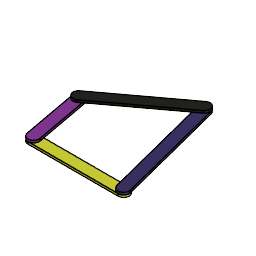
four_bar_linkage (Autodesk Fusion 360 design; units mm, degrees)
Autodesk Fusion 360 part; units mm, degrees
sketch "Sketch1" plane through (0, 0, 0) normal (0, 0, 1) x (1, 0, 0)
  line L0 (0, -5) -> (50, -5)
  arc A0 (50, -5) -> (50, 5) centre (50, 0) ccw
  line L1 (50, 5) -> (0, 5)
  arc A1 (0, 5) -> (0, -5) centre (0, 0) ccw
  line L2 (0, 0) -> (50, 0) construction
  line L3 (0, -25) -> (80, -25)
  arc A2 (80, -25) -> (80, -15) centre (80, -20) ccw
  line L4 (80, -15) -> (0, -15)
  arc A3 (0, -15) -> (0, -25) centre (0, -20) ccw
  line L5 (0, -20) -> (80, -20) construction
  line L6 (0, -45) -> (80, -45)
  arc A4 (80, -45) -> (80, -35) centre (80, -40) ccw
  line L7 (80, -35) -> (0, -35)
  arc A5 (0, -35) -> (0, -45) centre (0, -40) ccw
  line L8 (0, -40) -> (80, -40) construction
  line L9 (0, -65) -> (100, -65)
  arc A6 (100, -65) -> (100, -55) centre (100, -60) ccw
  line L10 (100, -55) -> (0, -55)
  arc A7 (0, -55) -> (0, -65) centre (0, -60) ccw
  line L11 (0, -60) -> (100, -60) construction
  dimension "d1" = 10
  dimension "d2" = 10
  dimension "d3" = 10
  dimension "d4" = 10
  constraint tangent L0 A0
  constraint tangent A0 L1
  constraint parallel L0 L1
  constraint tangent L1 A1
  constraint tangent L0 A1
  constraint horizontal L2
  constraint coincident A1.centre L2.start
  constraint tangent L3 A2
  constraint tangent A2 L4
  constraint parallel L3 L4
  constraint tangent L4 A3
  constraint tangent L3 A3
  constraint horizontal L5
  constraint tangent L6 A4
  constraint tangent A4 L7
  constraint parallel L6 L7
  constraint tangent L7 A5
  constraint tangent L6 A5
  constraint horizontal L8
  constraint tangent L9 A6
  constraint tangent A6 L10
  constraint parallel L9 L10
  constraint tangent L10 A7
  constraint tangent L9 A7
  constraint parallel L6 L11
  measures "d1" diameter of A0
  measures "d2" diameter of A2
  measures "d3" diameter of A4
  measures "d4" diameter of A6
extrude "Extrude1" add sketch "Sketch1" along normal blind 2 makes body 1 at (53.3333, -21.6667, 0) makes body 2 at (53.3333, -41.6667, 0) makes body 3 at (33.3333, -1.6667, 0) makes body 4 at (66.6667, -61.6667, 0) in component "Component"
copy_body "Body->Comp1" bodies 1 removing the originals makes body 5 in component "Component'"
copy_body "Body->Comp2" bodies 2 removing the originals makes body 6 in component "Component''"
copy_body "Body->Comp3" bodies 3 removing the originals makes body 7 in component "Component'''"
copy_body "Body->Comp4" bodies 4 removing the originals makes body 8 in component "Component''''"
component "Component" placed x (1, 0, 0) y (0, 1, 0) z (0, 0, 1) at (0, 0, 0)
component "Component'" placed x (1, 0, 0) y (0, 1, 0) z (0, 0, 1) at (0, 0, 0) in component "Component"
component "Component''" placed x (-0.724996, -0.688754, 0) y (0.688754, -0.724996, 0) z (0, 0, 1) at (38.6748, 23.4997, 4) in component "Component"
component "Component'''" placed x (-0.9375, 0.347985, 0) y (0.347985, 0.9375, 0) z (0, 0, -1) at (0, -20, 4) in component "Component"
component "Component''''" placed x (-0.688754, 0.724996, 0) y (0.724996, 0.688754, 0) z (0, 0, -1) at (123.4997, 21.3252, 4) in component "Component"
